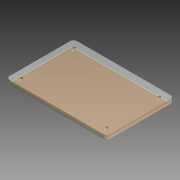
# Autodesk Inventor part: nanopc_t4_cover
Saved by Autodesk Inventor 2013 SP2 (Build 170200200, 200)
## iProperties
Created: 2018-09-03
Part Number: nanopc_t4_cover
Material: Acrylic
Document SubType Name: Modeling
Designer: alex
Density: 1.188 g/cm^3
Author: alex
Autodesk Inventor part; units mm, degrees
ref_plane "YZ Plane" through (0, 0, 0) normal (1, 0, 0) x (0, 1, 0)
ref_plane "XZ Plane" through (0, 0, 0) normal (0, 1, 0) x (-1, 0, 0)
ref_plane "XY Plane" through (0, 0, 0) normal (0, 0, 1) x (1, 0, 0)
ref_plane "Work Plane1" through (0, 0, 0) normal (0, 0, 1) x (1, 0, 0)
sketch "Sketch1" plane through (0, 0, 0) normal (0, 0, 1) x (1, 0, 0)
  line L0 (-4.2, 67.6475) -> (97.8, 67.6475)
  line L1 (101.8, 63.6475) -> (101.8, -2.3525)
  line L2 (97.8, -6.3525) -> (-4.2, -6.3525)
  line L3 (-8.2, -2.3525) -> (-8.2, 63.6475)
  circle A0 centre (0, 59.4475) radius 1.6 projected
  circle A1 centre (93.6, 59.4475) radius 1.6 projected
  circle A2 centre (93.6, 1.8475) radius 1.6 projected
  circle A3 centre (0, 1.8475) radius 1.6 projected
  arc A4 (-4.2, 67.6475) -> (-8.2, 63.6475) centre (-4.2, 63.6475) ccw
  arc A5 (-8.2, -2.3525) -> (-4.2, -6.3525) centre (-4.2, -2.3525) ccw
  arc A6 (97.8, -6.3525) -> (101.8, -2.3525) centre (97.8, -2.3525) ccw
  arc A7 (101.8, 63.6475) -> (97.8, 67.6475) centre (97.8, 63.6475) ccw
  point P0 (0, 0)
  point P1 (101.8, -6.3525)
  point P2 (101.8, 67.6475)
  point P3 (-8.2, -6.3525)
  dimension "d0" = 74
  dimension "d2" = 110
  dimension "d3" = 4
  constraints: 8 end point, 8 point on circle, 8 tangent, 6 point on line, 4 centre point, 3 equal radius, 2 parallel, 1 horizontal, 1 perpendicular
  measures "d0" distance of point (101.8, 67.648) point (101.8, -6.352)
  measures "d2" distance of point (101.8, -6.352) point (-8.2, -6.352)
  measures "d3" radius of A4
extrude "Extrusion1" add sketch "Sketch1" along normal blind 4.7
body "Solid1"
